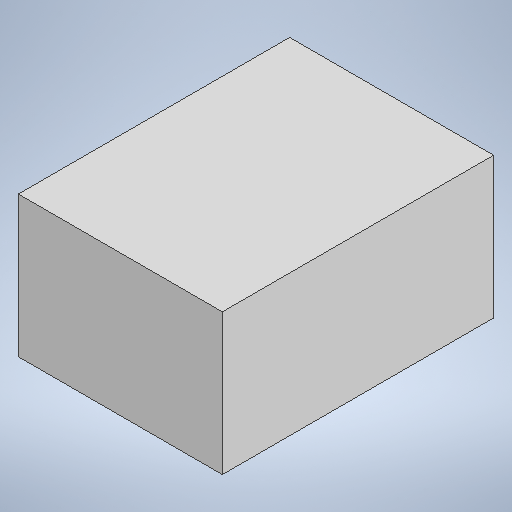
# Autodesk Inventor part: INTERNALCOMPONENTSPLACEHOLDER
Saved by Autodesk Inventor 2025.2 (Build 292293000, 293)
## iProperties
Created: 2025-01-28
Part Number: INTERNALCOMPONENTSPLACEHOLDER
Material: Generic
Document SubType Name: Modeling
Designer: cbast
Density: 1 g/cm^3
Appearance: Default
Author: cbast
Autodesk Inventor part; units mm, degrees
ref_plane "YZ Plane" through (0, 0, 0) normal (1, 0, 0) x (0, 1, 0)
ref_plane "XZ Plane" through (0, 0, 0) normal (0, 1, 0) x (-1, 0, 0)
ref_plane "XY Plane" through (0, 0, 0) normal (0, 0, 1) x (1, 0, 0)
sketch "Sketch1" plane through (0, 0, 0) normal (0, 1, 0) x (-1, 0, 0)
  line L0 (-81.2, 107.976) -> (81.2, 107.976)
  line L1 (81.2, 107.976) -> (81.2, -107.976)
  line L2 (81.2, -107.976) -> (-81.2, -107.976)
  line L3 (-81.2, -107.976) -> (-81.2, 107.976)
  line L4 (-81.2, 107.976) -> (81.2, -107.976) construction
  line L5 (81.2, 107.976) -> (-81.2, -107.976) construction
  point P0 (0, 0)
  dimension "d0" = 162.4
  dimension "d1" = 215.952
  constraints: 12 end point, 2 midpoint, 2 parallel, 1 horizontal, 1 perpendicular
  measures "d0" distance of L1.end L2.end
  measures "d1" distance of L0.end L1.end
extrude "Extrusion1" add sketch "Sketch1" along normal blind 112.2
body "Solid1"
